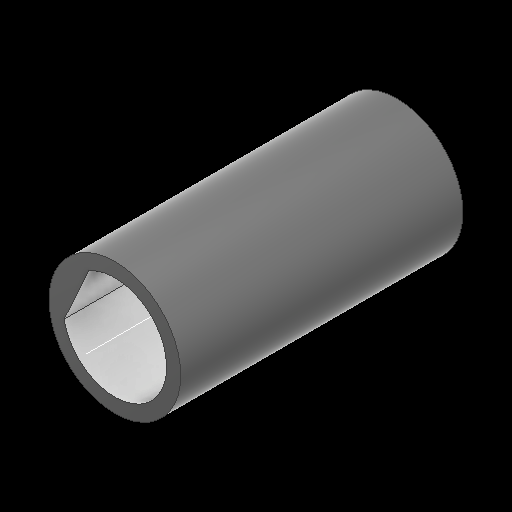
# Autodesk Inventor part: RobotWheelMK1printtest
Saved by Autodesk Inventor 2025 (Build 290162000, 162)
## iProperties
Created: 2024-11-18
Part Number: RobotWheelMK1printtest
Material: Generic
Document SubType Name: Modeling
Designer: Trevor
Density: 1 g/cm^3
Appearance: Default
Author: Trevor
Autodesk Inventor part; units mm, degrees
ref_plane "YZ Plane" through (0, 0, 0) normal (1, 0, 0) x (0, 1, 0)
ref_plane "XZ Plane" through (0, 0, 0) normal (0, 1, 0) x (-1, 0, 0)
sketch "Sketch1" plane through (0, 0, 0) normal (0, 0, 1) x (1, 0, 0)
  line L0 (-2.4408, -0.5408) -> (-1.2026, 2.1918) projected
  arc A0 (-2.4408, -0.5408) -> (-1.2026, 2.1918) centre (0, 0) ccw projected
  circle A1 centre (0, 0) radius 3.5
  line L1 (-3.6608, -0.2297) -> (-3.4925, -0.2297)
  line L2 (-3.4925, 0.2297) -> (-3.6608, 0.2297)
  line L3 (-3.6608, 0.2297) -> (-3.6608, -0.2297)
  line L4 (-3.6608, -0.2297) -> (-3.5, 0) construction
  line L5 (-3.5, 0) -> (-3.6608, 0.2297) construction
  point P0 (0, 0)
  dimension "d0" = 7
  constraints: 10 end point, 3 point on circle, 1 centre point, 1 coincident, 1 horizontal, 1 parallel
  measures "d0" diameter of A1
ref_plane "Work Plane1" through (-2, -2, 15) normal (0, 0, 1) x (1, 0, 0)
extrude "Extrusion1" add sketch "Sketch1" along normal up to surface (15 mm away) contours A1
sketch "Sketch2" plane through (0, 0, 15) normal (0, 0, 1) x (1, 0, 0)
  arc A0 (-2.4408, -0.5408) -> (-1.2026, 2.1918) centre (0, 0) ccw projected
  line L0 (-1.2026, 2.1918) -> (-2.4408, -0.5408) projected
  circle A1 centre (0, 0) radius 3.5 projected
  arc A2 (-2.702, -0.5115) -> (-1.3968, 2.3688) centre (0, 0) ccw
  line L1 (-2.702, -0.5115) -> (-1.3968, 2.3688)
  point P0 (0, 0)
  dimension "d9" = 0.25
  constraints: 2 end point, 2 point on circle, 1 centre point, 1 other
  measures "d9" radial gap between concentric circles of A0 A2
extrude "Extrusion2" cut sketch "Sketch2" against normal up to surface (15 mm away) contours L1 A2
body "Solid1"
